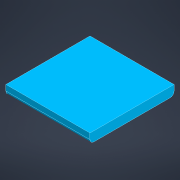
# Autodesk Inventor part: BottomSeatCushion
Saved by Autodesk Inventor 2021 (Build 250183000, 183)
## iProperties
Created: 2021-01-30
Part Number: BottomSeatCushion
Material: Generic
Document SubType Name: Modeling
Designer: argon
Density: 1 g/cm^3
Appearance: Sky Blue Medium
Author: argon
Autodesk Inventor part; units mm, degrees
ref_plane "YZ Plane" through (0, 0, 0) normal (1, 0, 0) x (0, 1, 0)
ref_plane "XZ Plane" through (0, 0, 0) normal (0, 1, 0) x (-1, 0, 0)
ref_plane "XY Plane" through (0, 0, 0) normal (0, 0, 1) x (1, 0, 0)
sketch "Sketch1" plane through (0, 0, 0) normal (0, 1, 0) x (-1, 0, 0)
  line L0 (220, 220) -> (-220, 220)
  line L1 (-220, 220) -> (-220, -220)
  line L2 (-220, -220) -> (220, -220)
  line L3 (220, -220) -> (220, 220)
  line L4 (220, 220) -> (-220, -220) construction
  line L5 (-220, 220) -> (220, -220) construction
  point P0 (0, 0)
  dimension "d0" = 440
  dimension "d1" = 440
  constraints: 12 end point, 2 midpoint, 2 parallel, 1 horizontal, 1 perpendicular
  measures "d0" distance of L0.end L1.end
  measures "d1" distance of L1.end L2.end
extrude "Extrusion1" add sketch "Sketch1" along normal blind 50
fillet "Fillet1" radius 20 2 edges at (0, 0, 220) (0, 0, -220)
body "Solid1"
